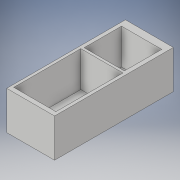
# Autodesk Inventor part: collector
Saved by Autodesk Inventor 2019 (Build 230136000, 136)
## iProperties
Created: 2020-02-18
Part Number: collector
Material: Generic
Document SubType Name: Modeling
Designer: Dell
Density: 1 g/cm^3
Appearance: Default
Author: Dell
Autodesk Inventor part; units mm, degrees
ref_plane "YZ Plane" through (0, 0, 0) normal (1, 0, 0) x (0, 1, 0)
ref_plane "XZ Plane" through (0, 0, 0) normal (0, 1, 0) x (-1, 0, 0)
ref_plane "XY Plane" through (0, 0, 0) normal (0, 0, 1) x (1, 0, 0)
sketch "Sketch1" plane through (0, 0, 0) normal (0, 1, 0) x (-1, 0, 0)
  line L0 (144.8249, 258.4464) -> (-105.1751, 258.4464)
  line L1 (-105.1751, 258.4464) -> (-105.1751, -361.5536)
  line L2 (-105.1751, -361.5536) -> (144.8249, -361.5536)
  line L3 (144.8249, -361.5536) -> (144.8249, 258.4464)
  point P0 (0, 0)
  dimension "d0" = 620
  dimension "d1" = 250
  constraints: 8 end point, 2 parallel, 1 horizontal, 1 perpendicular
  measures "d0" distance of L2.end L0.start
  measures "d1" distance of L1.end L2.end
extrude "Extrusion1" add sketch "Sketch1" along normal blind 200
sketch "Sketch2" plane through (0, 200, 0) normal (0, 1, 0) x (1, 0, 0)
  line L0 (89.2369, -235.4618) -> (-130.7631, -235.4618)
  line L1 (-130.7631, -235.4618) -> (-130.7631, 114.5382)
  line L2 (-130.7631, 114.5382) -> (89.2369, 114.5382)
  line L3 (89.2369, 114.5382) -> (89.2369, -235.4618)
  point P0 (0, 0)
  dimension "d4" = 220
  dimension "d5" = 350
  constraints: 8 end point, 2 parallel, 1 horizontal, 1 perpendicular
  measures "d4" distance of L0.start L0.end
  measures "d5" distance of L2.end L0.start
extrude "Extrusion2" cut sketch "Sketch2" against normal blind 185
sketch "Sketch3" plane through (0, 200, 0) normal (0, 1, 0) x (1, 0, 0)
  line L0 (-126.25, 127.5) -> (83.75, 127.5)
  line L1 (83.75, 127.5) -> (83.75, 322.5)
  line L2 (83.75, 322.5) -> (-126.25, 322.5)
  line L3 (-126.25, 322.5) -> (-126.25, 127.5)
  point P0 (0, 0)
  dimension "d8" = 210
  dimension "d9" = 195
  constraints: 8 end point, 2 parallel, 1 horizontal, 1 perpendicular
  measures "d8" distance of L1.end L2.end
  measures "d9" distance of L2.end L0.start
extrude "Extrusion3" cut sketch "Sketch3" against normal blind 185
body "Solid1"
